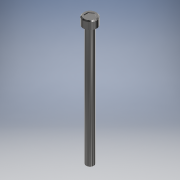
# Autodesk Inventor part: bolt
Saved by Autodesk Inventor 2018 (Build 220112000, 112)
## iProperties
Created: 2023-12-05
Part Number: bolt
Material: Generic
Document SubType Name: Modeling
Designer: DDUGKY
Density: 1 g/cm^3
Appearance: Steel - Polished
Author: DDUGKY
Autodesk Inventor part; units mm, degrees
ref_plane "YZ Plane" through (0, 0, 0) normal (1, 0, 0) x (0, 1, 0)
ref_plane "XZ Plane" through (0, 0, 0) normal (0, 1, 0) x (-1, 0, 0)
ref_plane "XY Plane" through (0, 0, 0) normal (0, 0, 1) x (1, 0, 0)
sketch "Sketch1" plane through (0, 0, 0) normal (0, 0, 1) x (1, 0, 0)
  circle A0 centre (0, 0) radius 3.5
  dimension "d0" = 7
  constraints: 1 centre point, 1 coincident
  measures "d0" diameter of A0
extrude "Extrusion1" add sketch "Sketch1" along normal blind 4
sketch "Sketch2" plane through (0, 0, 0) normal (0, 0, 1) x (1, 0, 0)
  circle A0 centre (0, 0) radius 2
  dimension "d3" = 4
  constraints: 1 centre point, 1 coincident
  measures "d3" diameter of A0
extrude "Extrusion2" add sketch "Sketch2" against normal blind 62
chamfer "Chamfer1" distance 0.5 angle 45 2 edges at (-3.5, 0, 4) (-2, 0, -62)
sketch "Sketch3" plane through (0, 0, 4) normal (0, 0, 1) x (1, 0, 0)
  circle A0 centre (0, 0) radius 2 projected
  line L0 (-2, 1.1547) -> (0, 2.3094)
  line L1 (0, 2.3094) -> (2, 1.1547)
  line L2 (2, 1.1547) -> (2, -1.1547)
  line L3 (2, -1.1547) -> (0, -2.3094)
  line L4 (0, -2.3094) -> (-2, -1.1547)
  line L5 (-2, -1.1547) -> (-2, 1.1547)
  point P0 (-2, 0)
  constraints: 12 end point, 1 coincident, 1 horizontal alignment, 1 midpoint, 14 other
extrude "Extrusion3" cut sketch "Sketch3" against normal blind 0.5
body "Solid1"
